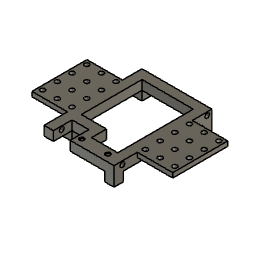
Trolley Base Assembly (Autodesk Fusion 360 design; units mm, degrees)
Autodesk Fusion 360 part; units mm, degrees
sketch "Sketch1" plane through (0, 0, 0) normal (0, 0, 1) x (1, 0, 0)
  line L0 (0, 0) -> (75, 0)
  line L1 (75, 0) -> (75, 100)
  line L2 (75, 100) -> (0, 100)
  line L3 (0, 100) -> (0, 0)
  line L4 (10, 90) -> (65, 90)
  line L5 (65, 90) -> (65, 10)
  line L6 (65, 10) -> (10, 10)
  line L7 (10, 10) -> (10, 90)
  dimension "d1" = 75
  dimension "d2" = 100
  dimension "d3" = 10
  dimension "d4" = 10
  dimension "d5" = 10
  dimension "d6" = 10
  constraint horizontal L0
  constraint vertical L1
  constraint horizontal L2
  constraint vertical L3
  constraint coincident L0.start L3.end
  constraint horizontal L4
  constraint vertical L5
  constraint horizontal L6
  constraint vertical L7
  measures "d1" distance of L1 L3
  measures "d2" distance of L0 L2
  measures "d3" distance of L0 L6
  measures "d4" distance of L1 L5
  measures "d5" distance of L2 L4
  measures "d6" distance of L3 L7
extrude "Extrude1" add sketch "Sketch1" along normal blind 10 makes body 1
sketch "Sketch2" plane through (0, 0, 0) normal (0, 0, -1) x (1, 0, 0)
  line L0 (10, -10) -> (65, -10)
  line L1 (65, -10) -> (65, -90)
  line L2 (65, -90) -> (10, -90)
  line L3 (10, -90) -> (10, -10)
  line L4 (0, 0) -> (0, -100)
  line L5 (0, -100) -> (75, -100)
  line L6 (75, -100) -> (75, 0)
  line L7 (75, 0) -> (0, 0)
  line L8 (10, -10) -> (0, -10)
  line L9 (0, -10) -> (0, 0)
  line L10 (0, 0) -> (10, 0)
  line L11 (10, 0) -> (10, -10)
  line L12 (65, -10) -> (75, -10)
  line L13 (75, -10) -> (75, 0)
  line L14 (75, 0) -> (65, 0)
  line L15 (65, 0) -> (65, -10)
  line L16 (65, -90) -> (75, -90)
  line L17 (75, -90) -> (75, -100)
  line L18 (75, -100) -> (65, -100)
  line L19 (65, -100) -> (65, -90)
  line L20 (0, -90) -> (10, -90)
  line L21 (10, -90) -> (10, -100)
  line L22 (10, -100) -> (0, -100)
  line L23 (0, -100) -> (0, -90)
  constraint horizontal L8
  constraint vertical L9
  constraint horizontal L10
  constraint vertical L11
  constraint coincident L4.start L7.end
  constraint coincident L0.start L3.end
  constraint horizontal L12
  constraint vertical L13
  constraint horizontal L14
  constraint vertical L15
  constraint coincident L6.end L7.start
  constraint coincident L0.end L1.start
  constraint horizontal L16
  constraint vertical L17
  constraint horizontal L18
  constraint vertical L19
  constraint coincident L5.end L6.start
  constraint coincident L1.end L2.start
  constraint horizontal L20
  constraint vertical L21
  constraint horizontal L22
  constraint vertical L23
  constraint coincident L5 L21.end
extrude "Extrude2" add sketch "Sketch2" along normal blind 10 contours L4 L7 L8 L9 L10 L11 | L6 L7 L12 L13 L14 L15 | L4 L5 L20 L21 L22 L23 | L5 L6 L16 L17 L18 L19 bodies 1
sketch "Sketch3" plane through (75, 0, 0) normal (1, 0, 0) x (0, 1, 0)
  line L0 (10, 0) -> (90, 0)
  line L1 (90, 0) -> (90, -10)
  line L2 (90, -10) -> (100, -10)
  line L3 (100, -10) -> (100, 10)
  line L4 (100, 10) -> (0, 10)
  line L5 (0, 10) -> (0, -10)
  line L6 (0, -10) -> (10, -10)
  line L7 (10, -10) -> (10, 0)
  circle A0 centre (5, 5) radius 2.5
  circle A1 centre (95, 5) radius 2.5
  dimension "d11" = 5
  dimension "d12" = 5
  dimension "d13" = 5
  dimension "d14" = 5
  dimension "d15" = 5
  dimension "d16" = 5
  measures "d11" diameter of A1
  measures "d12" diameter of A0
  measures "d13" distance of L4 A1.centre
  measures "d14" distance of L3 A1.centre
  measures "d15" distance of L4 A0.centre
  measures "d16" distance of L5 A0.centre
extrude "Extrude3" cut sketch "Sketch3" against normal blind 80 contours A0 | A1 bodies 1
sketch "Sketch4" plane through (0, 0, 0) normal (0, 0, -1) x (1, 0, 0)
  line L0 (10, 0) -> (10, -10)
  line L1 (10, -10) -> (65, -10)
  line L2 (65, -10) -> (65, 0)
  line L3 (65, 0) -> (10, 0)
  circle A0 centre (33, -5) radius 2.5
  circle A1 centre (61, -5) radius 2.5
  line L4 (10, -10) -> (10, -90)
  line L5 (65, -90) -> (65, -10)
  line L6 (10, -50) -> (65, -50)
  circle A2 centre (61, -95) radius 2.5
  circle A3 centre (33, -95) radius 2.5
  dimension "d19" = 5
  dimension "d20" = 23
  dimension "d21" = 5
  dimension "d22" = 4
  dimension "d23" = 5
  dimension "d24" = 5
  constraint midpoint L4 L6.start
  constraint midpoint L5 L6.end
  constraint symmetric A0 L6 A3
  constraint symmetric A1 L6 A2
  measures "d19" diameter of A0
  measures "d20" distance of L0 A0.centre
  measures "d21" diameter of A1
  measures "d22" distance of L2 A1.centre
  measures "d23" distance of L1 A1.centre
  measures "d24" diameter of A0
extrude "Extrude4" cut sketch "Sketch4" against normal blind 12 contours A0 | A1 bodies 1
extrude "Extrude5" cut sketch "Sketch4" against normal blind 12 contours A2 | A3 bodies 1
sketch "Sketch6" plane through (0, 0, 10) normal (0, 0, 1) x (-1, 0, 0)
  circle A0 centre (-33, -95) radius 2.5
  circle A1 centre (-61, -95) radius 2.5
  circle A2 centre (-33, -5) radius 2.5
  circle A3 centre (-61, -5) radius 2.5
  line L0 (-65, -10) -> (-10, -10)
  line L1 (-10, -10) -> (-10, -90)
  line L2 (-10, -90) -> (-65, -90)
  line L3 (-65, -90) -> (-65, -10)
  line L4 (0, -100) -> (0, 0)
  line L5 (0, 0) -> (-75, 0)
  line L6 (-75, 0) -> (-75, -100)
  line L7 (-75, -100) -> (0, -100)
  line L8 (-75, -80) -> (-105, -80)
  line L9 (-105, -80) -> (-105, -20)
  line L10 (-105, -20) -> (-75, -20)
  line L11 (-75, -20) -> (-75, -80)
  line L12 (-37.5, -10) -> (-37.5, -90)
  line L13 (30, -20) -> (0, -20)
  line L14 (0, -80) -> (30, -80)
  line L15 (0, -20) -> (0, -80)
  line L16 (30, -80) -> (30, -20)
  dimension "d32" = 30
  dimension "d33" = 20
  dimension "d34" = 20
  constraint horizontal L8
  constraint vertical L9
  constraint horizontal L10
  constraint vertical L11
  constraint coincident L6 L8.start
  constraint midpoint L0 L12.start
  constraint midpoint L2 L12.end
  constraint symmetric L8.start L12 L14.start
  constraint symmetric L8.end L12 L14.end
  constraint symmetric L9.end L12 L13.start
  constraint symmetric L10.end L12 L13.end
  measures "d32" distance of L9 L11
  measures "d33" distance of L5 L10
  measures "d34" distance of L7 L8
extrude "Extrude6" add sketch "Sketch6" against normal blind 5 contours L4 L13 L14 L15 L16 | L6 L8 L9 L10 L11 bodies 1
sketch "Sketch7" plane through (0, 0, 10) normal (0, 0, 1) x (-1, 0, 0)
  circle A0 centre (-33, -95) radius 2.5
  circle A1 centre (-61, -95) radius 2.5
  circle A2 centre (-33, -5) radius 2.5
  circle A3 centre (-61, -5) radius 2.5
  line L0 (-65, -10) -> (-10, -10)
  line L1 (-10, -10) -> (-10, -90)
  line L2 (-10, -90) -> (-65, -90)
  line L3 (-65, -90) -> (-65, -10)
  line L4 (0, -100) -> (0, -80)
  line L5 (0, -80) -> (30, -80)
  line L6 (30, -80) -> (30, -20)
  line L7 (30, -20) -> (0, -20)
  line L8 (0, -20) -> (0, 0)
  line L9 (0, 0) -> (-75, 0)
  line L10 (-75, 0) -> (-75, -20)
  line L11 (-75, -20) -> (-105, -20)
  line L12 (-105, -20) -> (-105, -80)
  line L13 (-105, -80) -> (-75, -80)
  line L14 (-75, -80) -> (-75, -100)
  line L15 (-75, -100) -> (0, -100)
  line L16 (0, -20) -> (-28, -20)
  line L17 (-28, -20) -> (-28, 0)
  line L18 (-28, 0) -> (0, 0)
  line L19 (0, 0) -> (0, -20)
  dimension "d37" = 28
  constraint horizontal L16
  constraint vertical L17
  constraint horizontal L18
  constraint vertical L19
  constraint coincident L9 L17.end
  constraint coincident L7.end L8.start
  measures "d37" distance of L17 L19
extrude "Extrude7" cut sketch "Sketch7" against normal blind 20 contours L0 L1 L8 L9 L16 L17 L18 L19 | L0 L1 L16 L17 bodies 1
sketch "Sketch8" plane through (0, 0, 10) normal (0, 0, 1) x (-1, 0, 0)
  line L0 (30, -20) -> (-10, -20)
  line L1 (-10, -20) -> (-10, -90)
  line L2 (-10, -90) -> (-65, -90)
  line L3 (-65, -90) -> (-65, -10)
  line L4 (-65, -10) -> (-28, -10)
  line L5 (-28, -10) -> (-28, 0)
  line L6 (-28, 0) -> (-75, 0)
  line L7 (-75, 0) -> (-75, -20)
  line L8 (-75, -20) -> (-105, -20)
  line L9 (-105, -20) -> (-105, -80)
  line L10 (-105, -80) -> (-75, -80)
  line L11 (-75, -80) -> (-75, -100)
  line L12 (-75, -100) -> (0, -100)
  line L13 (0, -100) -> (0, -80)
  line L14 (0, -80) -> (30, -80)
  line L15 (30, -80) -> (30, -20)
  circle A0 centre (-33, -95) radius 2.5
  circle A1 centre (-61, -95) radius 2.5
  circle A2 centre (-33, -5) radius 2.5
  circle A3 centre (-61, -5) radius 2.5
  line L16 (-10, -20) -> (-28, -20)
  line L17 (-36.8946, -30) -> (-10, -30)
  line L18 (-10, -30) -> (-10, -20)
  line L19 (-28, -10) -> (-36.8946, -10)
  line L20 (-36.8946, -10) -> (-36.8946, -20)
  line L21 (-28, -20) -> (-28, -10)
  line L22 (-36.8946, -20) -> (-36.8946, -30)
  dimension "d40" = 10
  constraint horizontal L16
  constraint horizontal L17
  constraint vertical L18
  constraint coincident L0.end L1.start
  constraint horizontal L19
  constraint vertical L20
  constraint vertical L21
  constraint coincident L4.end L5.start
  constraint perpendicular L17 L22
  measures "d40" distance of L16 L17
extrude "Extrude8" add sketch "Sketch8" against normal blind 10 contours L1 L4 L16 L17 L18 L19 L20 L21 L22 bodies 1
sketch "Sketch9" plane through (0, 0, 0) normal (0, 0, -1) x (1, 0, 0)
  circle A0 centre (61, -5) radius 2.5
  circle A1 centre (33, -5) radius 2.5
  line L0 (28, -20) -> (0, -20)
  line L1 (0, -20) -> (0, -90)
  line L2 (0, -90) -> (10, -90)
  line L3 (10, -90) -> (10, -30)
  line L4 (10, -30) -> (36.8946, -30)
  line L5 (36.8946, -30) -> (36.8946, -10)
  line L6 (36.8946, -10) -> (65, -10)
  line L7 (65, -10) -> (65, 0)
  line L8 (65, 0) -> (28, 0)
  line L9 (28, 0) -> (28, -20)
  line L10 (0, -20) -> (10, -20)
  line L11 (10, -20) -> (10, -30)
  line L12 (10, -30) -> (0, -30)
  line L13 (0, -30) -> (0, -20)
  constraint horizontal L10
  constraint vertical L11
  constraint horizontal L12
  constraint vertical L13
  constraint coincident L3.end L4.start
  constraint coincident L0.end L1.start
extrude "Extrude9" add sketch "Sketch9" along normal blind 10 contours L0 L1 L10 L11 L12 L13 bodies 1
sketch "Sketch10" plane through (0, 0, 10) normal (0, 0, 1) x (-1, 0, 0)
  line L0 (-10, -30) -> (-10, -90)
  line L1 (-10, -90) -> (-65, -90)
  line L2 (-65, -90) -> (-65, -10)
  line L3 (-65, -10) -> (-36.8946, -10)
  line L4 (-36.8946, -10) -> (-36.8946, -30)
  line L5 (-36.8946, -30) -> (-10, -30)
  line L6 (30, -20) -> (-28, -20)
  line L7 (-28, -20) -> (-28, 0)
  line L8 (-28, 0) -> (-75, 0)
  line L9 (-75, 0) -> (-75, -20)
  line L10 (-75, -20) -> (-105, -20)
  line L11 (-105, -20) -> (-105, -80)
  line L12 (-105, -80) -> (-75, -80)
  line L13 (-75, -80) -> (-75, -100)
  line L14 (-75, -100) -> (0, -100)
  line L15 (0, -100) -> (0, -80)
  line L16 (0, -80) -> (30, -80)
  line L17 (30, -80) -> (30, -20)
  circle A0 centre (-33, -95) radius 2.5
  circle A1 centre (-61, -95) radius 2.5
  circle A2 centre (-33, -5) radius 2.5
  circle A3 centre (-61, -5) radius 2.5
  line L18 (-30, -100) -> (-37.5, -100)
  line L19 (-37.5, -100) -> (-37.5, -90)
  line L20 (-37.5, -90) -> (-30, -90)
  line L21 (-30, -90) -> (-30, -100)
  constraint horizontal L18
  constraint vertical L19
  constraint horizontal L20
  constraint vertical L21
  constraint midpoint L1 L19.end
  constraint coincident L14 L18.start
extrude "Extrude10" add sketch "Sketch10" against normal blind 10 contours L1 L14 L18 L19 L20 L21 | A0 bodies 1
sketch "Sketch11" plane through (0, 0, 10) normal (0, 0, 1) x (-1, 0, 0)
  line L0 (-75, -100) -> (0, -100)
  line L1 (0, -100) -> (0, -80)
  line L2 (0, -80) -> (30, -80)
  line L3 (30, -80) -> (30, -20)
  line L4 (30, -20) -> (-28, -20)
  line L5 (-28, -20) -> (-28, 0)
  line L6 (-28, 0) -> (-75, 0)
  line L7 (-75, 0) -> (-75, -20)
  line L8 (-75, -20) -> (-105, -20)
  line L9 (-105, -20) -> (-105, -80)
  line L10 (-105, -80) -> (-75, -80)
  line L11 (-75, -80) -> (-75, -100)
  line L12 (-10, -90) -> (-65, -90)
  line L13 (-65, -90) -> (-65, -10)
  line L14 (-65, -10) -> (-36.8946, -10)
  line L15 (-36.8946, -10) -> (-36.8946, -30)
  line L16 (-36.8946, -30) -> (-10, -30)
  line L17 (-10, -30) -> (-10, -90)
  circle A0 centre (-61, -95) radius 2.5
  circle A1 centre (-33, -5) radius 2.5
  circle A2 centre (-61, -5) radius 2.5
  circle A3 centre (-45.25, -95) radius 2.5
  line L18 (-37.375, -90) -> (-37.375, -100)
  circle A4 centre (-29.5, -95) radius 2.5
  circle A5 centre (-13.75, -95) radius 2.5
  line L19 (-10, -87.125) -> (-65, -87.125)
  circle A6 centre (-13.75, -79.25) radius 2.5
  circle A7 centre (-29.5, -79.25) radius 2.5
  circle A8 centre (-45.25, -79.25) radius 2.5
  circle A9 centre (-61, -79.25) radius 2.5
  line L20 (-10, -71.375) -> (-65, -71.375)
  circle A10 centre (-13.75, -63.5) radius 2.5
  circle A11 centre (-13.75, -47.75) radius 2.5
  circle A12 centre (-29.5, -63.5) radius 2.5
  circle A13 centre (-29.5, -47.75) radius 2.5
  circle A14 centre (-45.25, -63.5) radius 2.5
  circle A15 centre (-61, -63.5) radius 2.5
  circle A16 centre (-61, -47.75) radius 2.5
  circle A17 centre (-45.25, -47.75) radius 2.5
  line L21 (-149.6879, -20) -> (-149.6879, -100)
  line L22 (-10, -39.875) -> (-65, -39.875)
  circle A18 centre (-13.75, -32) radius 2.5
  circle A19 centre (-29.5, -32) radius 2.5
  circle A20 centre (-45.25, -32) radius 2.5
  circle A21 centre (-61, -32) radius 2.5
  circle A22 centre (-13.75, -16.25) radius 2.5
  circle A23 centre (-285.6257, -32) radius 2.5
  circle A24 centre (-285.6257, -47.75) radius 2.5
  circle A25 centre (-269.8757, -47.75) radius 2.5
  circle A26 centre (-269.8757, -32) radius 2.5
  circle A27 centre (-269.8757, -63.5) radius 2.5
  circle A28 centre (-285.6257, -63.5) radius 2.5
  circle A29 centre (-254.1257, -32) radius 2.5
  circle A30 centre (-254.1257, -47.75) radius 2.5
  circle A31 centre (-254.1257, -63.5) radius 2.5
  line L23 (-75, 0) -> (-65, 0)
  line L24 (-65, -100) -> (-75, -100)
  line L25 (-75, -10) -> (-65, -10)
  line L26 (-68.875, -100) -> (-68.875, -10)
  circle A32 centre (-76.75, -47.75) radius 2.5
  circle A33 centre (-76.75, -32) radius 2.5
  circle A34 centre (-92.5, -32) radius 2.5
  circle A35 centre (-92.5, -63.5) radius 2.5
  circle A36 centre (-92.5, -47.75) radius 2.5
  circle A37 centre (-76.75, -63.5) radius 2.5
  circle A38 centre (-108.25, -32) radius 2.5
  circle A39 centre (-108.25, -47.75) radius 2.5
  circle A40 centre (-108.25, -63.5) radius 2.5
  circle A41 centre (-108.25, -79.25) radius 2.5
  circle A42 centre (-92.5, -79.25) radius 2.5
  circle A43 centre (-76.75, -79.25) radius 2.5
  circle A44 centre (-285.6257, -79.25) radius 2.5
  circle A45 centre (-269.8757, -79.25) radius 2.5
  circle A46 centre (-254.1257, -79.25) radius 2.5
  line L27 (-5.875, -20) -> (-5.875, -95)
  circle A47 centre (2, -79.25) radius 2.5
  circle A48 centre (17.75, -79.25) radius 2.5
  circle A49 centre (17.75, -63.5) radius 2.5
  circle A50 centre (2, -63.5) radius 2.5
  circle A51 centre (17.75, -47.75) radius 2.5
  circle A52 centre (2, -47.75) radius 2.5
  circle A53 centre (2, -32) radius 2.5
  circle A54 centre (17.75, -32) radius 2.5
  circle A55 centre (33.5, -79.25) radius 2.5
  circle A56 centre (33.5, -63.5) radius 2.5
  circle A57 centre (33.5, -47.75) radius 2.5
  circle A58 centre (33.5, -32) radius 2.5
  line L28 (0, -97.5) -> (-75, -97.5)
  line L29 (-75, -100) -> (0, -100)
  circle A59 centre (-13.75, -100) radius 2.5
  circle A60 centre (-29.5, -100) radius 2.5
  circle A61 centre (-45.25, -100) radius 2.5
  circle A62 centre (-61, -100) radius 2.5
  dimension "d48" = 15.75
  dimension "d49" = 5
  dimension "d50" = 7.875
  dimension "d51" = 7.875
  dimension "d52" = 7.875
  dimension "d53" = 7.875
  dimension "d55" = 7.875
  dimension "d75" = 7.875
  dimension "d86" = 2.5
  constraint coincident L12 L18.start
  constraint coincident L0 L18.end
  constraint perpendicular L0 L18
  constraint symmetric A0 L18 A5
  constraint symmetric A3 L18 A4
  constraint coincident L17 L19.start
  constraint coincident L13 L19.end
  constraint perpendicular L13 L19
  constraint symmetric A0 L19 A9
  constraint symmetric A3 L19 A8
  constraint symmetric A4 L19 A7
  constraint symmetric A5 L19 A6
  constraint coincident L17 L20.start
  constraint coincident L13 L20.end
  constraint perpendicular L13 L20
  constraint symmetric A0 L20 A16
  constraint symmetric A3 L20 A17
  constraint symmetric A4 L20 A13
  constraint symmetric A5 L20 A11
  constraint symmetric A6 L20 A10
  constraint symmetric A7 L20 A12
  constraint symmetric A8 L20 A14
  constraint symmetric A9 L20 A15
  constraint coincident L4 L21.start
  constraint perpendicular L4 L21
  constraint coincident L17 L22.start
  constraint coincident L13 L22.end
  constraint perpendicular L13 L22
  constraint symmetric A10 L22 A22
  constraint symmetric A11 L22 A18
  constraint symmetric A13 L22 A19
  constraint symmetric A16 L22 A21
  constraint symmetric A17 L22 A20
  constraint symmetric A10 L21 A28
  constraint symmetric A11 L21 A24
  constraint symmetric A12 L21 A27
  constraint symmetric A13 L21 A25
  constraint symmetric A14 L21 A31
  constraint symmetric A17 L21 A30
  constraint symmetric L21 A18 A23
  constraint symmetric L21 A19 A26
  constraint symmetric L21 A20 A29
  constraint coincident L24 L26.start
  constraint coincident L25 L26.end
  constraint perpendicular L14 L26
  constraint symmetric A7 L26 A41
  constraint symmetric A8 L26 A42
  constraint symmetric A9 L26 A43
  constraint symmetric A12 L26 A40
  constraint symmetric A13 L26 A39
  constraint symmetric A14 L26 A35
  constraint symmetric A15 L26 A37
  constraint symmetric A16 L26 A32
  constraint symmetric A17 L26 A36
  constraint symmetric A19 L26 A38
  constraint symmetric A20 L26 A34
  constraint symmetric A21 L26 A33
  constraint symmetric A6 L21 A44
  constraint symmetric A7 L21 A45
  constraint symmetric A8 L21 A46
  constraint coincident L4 L27.start
  constraint perpendicular L4 L27
  constraint symmetric A6 L27 A47
  constraint symmetric A7 L27 A48
  constraint symmetric A8 L27 A55
  constraint symmetric A10 L27 A50
  constraint symmetric A11 L27 A52
  constraint symmetric A12 L27 A49
  constraint symmetric A13 L27 A51
  constraint symmetric A14 L27 A56
  constraint symmetric A17 L27 A57
  constraint symmetric A18 L27 A53
  constraint symmetric A19 L27 A54
  constraint symmetric A20 L27 A58
  constraint coincident L1 L28.start
  constraint coincident L11 L28.end
  constraint perpendicular L11 L28
  constraint symmetric A0 L28 A62
  constraint symmetric A3 L28 A61
  constraint symmetric A4 L28 A60
  constraint symmetric A5 L28 A59
  measures "d48" distance of A0.centre A3.centre
  measures "d49" diameter of A3
  measures "d50" distance of A3.centre L18
  measures "d51" distance of A4.centre L19
  measures "d52" distance of A7.centre L20
  measures "d53" distance of A13.centre L22
  measures "d55" distance of A16.centre L26
  measures "d75" distance of A6.centre L27
  measures "d86" distance of L28 L29
sketch "Sketch12" plane through (0, 0, 10) normal (0, 0, 1) x (-1, 0, 0)
  line L0 (-105, -20) -> (-113, -20)
  line L1 (-113, -20) -> (-113, -84)
  line L2 (-113, -84) -> (-105, -84)
  line L3 (-105, -84) -> (-105, -20)
  line L4 (-105, -80) -> (-75, -80)
  line L5 (-105, -84) -> (-75, -84)
  line L6 (-75, -84) -> (-75, -80)
  line L7 (-75, -80) -> (-105, -80)
  line L8 (-105, -80) -> (-105, -84)
  line L9 (-113, -20) -> (-75, -20)
  line L10 (-75, -20) -> (-75, -25)
  line L11 (-75, -25) -> (-113, -25)
  line L12 (-113, -25) -> (-113, -20)
  line L13 (-75, -80) -> (-75, -20)
  line L14 (30, -20) -> (38, -20)
  line L15 (38, -20) -> (38, -84)
  line L16 (38, -84) -> (30, -84)
  line L17 (30, -84) -> (30, -20)
  line L18 (0, -80) -> (30, -80)
  line L19 (30, -84) -> (0, -84)
  line L20 (0, -84) -> (0, -80)
  line L21 (0, -80) -> (30, -80)
  line L22 (30, -80) -> (30, -84)
  line L23 (38, -20) -> (0, -20)
  line L24 (0, -20) -> (0, -25)
  line L25 (0, -25) -> (38, -25)
  line L26 (38, -25) -> (38, -20)
  line L27 (0, -20) -> (0, -30)
  point P0 (-105, -20)
  point P1 (30, -20)
  dimension "d56" = 8
  dimension "d57" = 4
  dimension "d58" = 8
  dimension "d59" = 4
  dimension "d60" = 5
  constraint horizontal L0
  constraint vertical L1
  constraint horizontal L2
  constraint vertical L3
  constraint coincident P0 L0.start
  constraint horizontal L5
  constraint vertical L6
  constraint horizontal L7
  constraint vertical L8
  constraint coincident L4.end L6.end
  constraint horizontal L9
  constraint vertical L10
  constraint horizontal L11
  constraint vertical L12
  constraint coincident L10.end L13
  constraint horizontal L14
  constraint vertical L15
  constraint horizontal L16
  constraint vertical L17
  constraint coincident P1 L14.start
  constraint horizontal L19
  constraint vertical L20
  constraint horizontal L21
  constraint vertical L22
  constraint coincident L18.start L20.end
  constraint horizontal L23
  constraint vertical L24
  constraint horizontal L25
  constraint vertical L26
  constraint midpoint L24.end L27
  measures "d56" distance of L1 L3
  measures "d57" distance of L2 L4
  measures "d58" distance of L15 L17
  measures "d59" distance of L16 L18
  measures "d60" distance of L23 L25
extrude "Extrude11" add sketch "Sketch12" against normal blind 5 contours L1 L2 L3 L8 L11 | L3 L4 L5 L6 L7 L8 bodies 1
extrude "Extrude12" cut sketch "Sketch12" against normal blind 5 contours L0 L1 L3 L9 L11 L12 | L3 L9 L10 L11 L13 bodies 1
extrude "Extrude13" add sketch "Sketch12" against normal blind 5 contours L15 L16 L17 L22 L25 | L17 L18 L19 L20 L21 L22 bodies 1
extrude "Extrude14" cut sketch "Sketch12" against normal blind 5 contours L14 L15 L17 L23 L25 L26 | L17 L23 L24 L25 L27 bodies 1
extrude "Extrude15" cut sketch "Sketch11" against normal blind 10 contours A3 | A4 | A5 bodies 1
extrude "Extrude16" cut sketch "Sketch11" against normal blind 10 contours L10 L11 A43 | L10 L11 A43 | A32 | A33 | A37 bodies 1
extrude "Extrude17" cut sketch "Sketch11" against normal blind 5 contours L10 A42 | L10 A42 | A34 | A35 | A36 | A38 | A39 | A40 | A41 bodies 1
extrude "Extrude18" cut sketch "Sketch11" against normal blind 10 contours L1 L2 A47 | L1 L2 A47 | L2 A48 | L2 A48 | A49 | A50 | A51 | A52 | A53 | A54 | A55 | A56 | A57 | A58 bodies 1
sketch "Sketch13" plane through (75, 0, 0) normal (1, 0, 0) x (0, 1, 0)
  circle A0 centre (95, 5) radius 2.5
  line L0 (81.0354, 5) -> (81.0354, 0)
  line L1 (81.0354, 0) -> (90, 0)
  line L2 (90, 0) -> (90, -10)
  line L3 (90, -10) -> (100, -10)
  line L4 (100, -10) -> (100, 10)
  line L5 (100, 10) -> (84, 10)
  line L6 (84, 10) -> (84, 5)
  line L7 (84, 5) -> (81.0354, 5)
  circle A1 centre (95, 5) radius 2.5
  constraint concentric A0 A1
extrude "Extrude19" cut 1 faces at (37.5, 95.4167, 5.8298) along direction (1, 0, 0) blind -500 and the other way blind -500 on bodies 1 bodies 1
sketch "Sketch14" plane through (0, 20, 0) normal (0, -1, 0) x (1, 0, 0)
  line L0 (0, 10) -> (0, -10)
  line L1 (0, -10) -> (10, -10)
  line L2 (10, -10) -> (10, 0)
  line L3 (10, 0) -> (28, 0)
  line L4 (28, 0) -> (28, 10)
  line L5 (28, 10) -> (0, 10)
  line L6 (10, 0) -> (0, 0)
  line L7 (0, 0) -> (0, 10)
  line L8 (0, 10) -> (10, 10)
  line L9 (10, 10) -> (10, 0)
  constraint horizontal L6
  constraint vertical L7
  constraint horizontal L8
  constraint vertical L9
  constraint coincident L0.start L5.end
  constraint coincident L2.end L3.start
extrude "Extrude20" add sketch "Sketch14" along normal blind 20 contours L0 L5 L6 L7 L8 L9 bodies 1
sketch "Sketch15" plane through (28, 0, 0) normal (-1, 0, 0) x (0, -1, 0)
  line L0 (-20, 0) -> (0, 0)
  line L1 (0, 0) -> (0, 10)
  line L2 (0, 10) -> (-20, 10)
  line L3 (-20, 10) -> (-20, 0)
  circle A0 centre (-5, 5) radius 2.5
sketch "Sketch16" plane through (75, 0, 0) normal (1, 0, 0) x (0, 1, 0)
  line L0 (30.2146, 0) -> (30.2146, 5)
  line L1 (30.2146, 5) -> (25, 5)
  line L2 (25, 5) -> (25, 10)
  line L3 (25, 10) -> (0, 10)
  line L4 (0, 10) -> (0, -10)
  line L5 (0, -10) -> (10, -10)
  line L6 (10, -10) -> (10, 0)
  line L7 (10, 0) -> (30.2146, 0)
  circle A0 centre (5, 5) radius 2.5
  circle A1 centre (5, 5) radius 2.5
  constraint concentric A0 A1
extrude "Extrude21" cut sketch "Sketch16" against normal blind 500 contours A0 A1 bodies 1
sketch "Sketch17" plane through (0, 0, 0) normal (-1, 0, 0) x (0, -1, 0)
  circle A0 centre (-95, 5) radius 2.5
  line L0 (-80.75, 0) -> (-80.75, 5)
  line L1 (-80.75, 5) -> (-84, 5)
  line L2 (-84, 5) -> (-84, 10)
  line L3 (-84, 10) -> (-100, 10)
  line L4 (-100, 10) -> (-100, -10)
  line L5 (-100, -10) -> (-90, -10)
  line L6 (-90, -10) -> (-90, 0)
  line L7 (-90, 0) -> (-80.75, 0)
sketch "Sketch18" plane through (75, 0, 0) normal (1, 0, 0) x (0, 1, 0)
  circle A0 centre (95, 5) radius 2.5
  line L0 (81.0354, 5) -> (81.0354, 0)
  line L1 (81.0354, 0) -> (90, 0)
  line L2 (90, 0) -> (90, -10)
  line L3 (90, -10) -> (100, -10)
  line L4 (100, -10) -> (100, 10)
  line L5 (100, 10) -> (84, 10)
  line L6 (84, 10) -> (84, 5)
  line L7 (84, 5) -> (81.0354, 5)
  line L8 (90, 0) -> (100, 0)
  line L9 (97.5, 0) -> (97.5, 10)
  line L10 (100, -10) -> (100, 10)
  circle A1 centre (100, 5) radius 2.5
  line L11 (90, 0) -> (100, 0)
  line L12 (100, 0) -> (100, 10)
  line L13 (100, 10) -> (90, 10)
  line L14 (90, 10) -> (90, 0)
  line L15 (90, 0) -> (100, 0)
  line L16 (100, 0) -> (100, -10)
  line L17 (100, -10) -> (90, -10)
  line L18 (90, -10) -> (90, 0)
  line L19 (100, 10) -> (100, 0)
  line L20 (100, -10) -> (100, 0)
  line L21 (90, 10) -> (100, 10)
  line L22 (100, 10) -> (100, 0)
  line L23 (100, 0) -> (90, 0)
  line L24 (90, 0) -> (90, 10)
  line L25 (100, 10) -> (105, 10)
  line L26 (105, 10) -> (105, 0)
  line L27 (105, 0) -> (100, 0)
  line L28 (100, 0) -> (100, 10)
  line L29 (100, 0) -> (105, 0)
  line L30 (105, 0) -> (105, -10)
  line L31 (105, -10) -> (100, -10)
  line L32 (100, -10) -> (100, 0)
  line L33 (90, 0) -> (95, 0)
  line L34 (95, 0) -> (95, -10)
  line L35 (95, -10) -> (90, -10)
  line L36 (90, -10) -> (90, 0)
  dimension "d87" = 2.5
  constraint coincident L8 L9.start
  constraint coincident L5 L9.end
  constraint symmetric A0 L9 A1
  constraint horizontal L11
  constraint vertical L12
  constraint horizontal L13
  constraint vertical L14
  constraint coincident L4.end L5.start
  constraint coincident L1.end L2.start
  constraint horizontal L15
  constraint vertical L16
  constraint horizontal L17
  constraint vertical L18
  constraint coincident L3.end L4.start
  constraint vertical L19
  constraint vertical L20
  constraint horizontal L21
  constraint vertical L22
  constraint horizontal L23
  constraint vertical L24
  constraint horizontal L25
  constraint vertical L26
  constraint horizontal L27
  constraint vertical L28
  constraint horizontal L29
  constraint vertical L30
  constraint horizontal L31
  constraint vertical L32
  constraint horizontal L33
  constraint vertical L34
  constraint horizontal L35
  constraint vertical L36
  constraint midpoint L3 L34.end
  measures "d87" distance of L9 L10
extrude "Extrude22" add sketch "Sketch18" against normal blind 75 contours L4 L10 A1 L12 L19 L22 L28 | L4 L10 A1 L12 L19 L22 L25 L26 L27 L28 L29 picked at (100.8333, 5) bodies 1
extrude "Extrude23" add sketch "Sketch18" against normal blind 75 contours L4 L10 L16 L20 L27 L29 L30 L31 L32 bodies 1
extrude "Extrude24" cut sketch "Sketch18" against normal blind 75 contours L2 L3 L8 L11 L15 L17 L18 L23 L33 L34 L35 L36 bodies 1
sketch "Sketch19" plane through (0, 105, 0) normal (0, 1, 0) x (-1, 0, 0)
  line L0 (-75, 10) -> (-75, -10)
  line L1 (-75, -10) -> (0, -10)
  line L2 (0, -10) -> (0, 10)
  line L3 (0, 10) -> (-75, 10)
  line L4 (-65, -10) -> (-10, -10)
  line L5 (-10, -10) -> (-10, 0)
  line L6 (-10, 0) -> (-65, 0)
  line L7 (-65, 0) -> (-65, -10)
  point P0 (-65, -10)
  point P1 (-10, 0)
  constraint horizontal L4
  constraint vertical L5
  constraint horizontal L6
  constraint vertical L7
  constraint coincident P1 L5.end
  constraint coincident P0 L4.start
extrude "Extrude25" cut sketch "Sketch19" against normal blind 10 contours L1 L4 L5 L6 L7 bodies 1
extrude "Extrude26" cut sketch "Sketch18" against normal blind 75 contours L4 L10 A1 L12 L19 L22 L28 | L4 L10 A1 L12 L19 L22 L28 bodies 1
extrude "Extrude27" add sketch "Sketch18" against normal blind 75 separate body contours A0 makes body 2
extrude "Extrude28" cut sketch "Sketch11" against normal blind 10 contours A0 | A3 | A4 | A5 bodies 2
sketch "Sketch20" plane through (75, 0, 0) normal (1, 0, 0) x (0, 1, 0)
  circle A0 centre (95, 5) radius 2.5
  circle A1 centre (95, 5) radius 2.5
  constraint concentric A0 A1
extrude "Extrude29" add sketch "Sketch20" against normal blind 75 bodies 2 1
sketch "Sketch21" plane through (0, 0, 0) normal (0, 1, 0) x (1, 0, 0)
sketch "Sketch22" plane through (0, 0, 10) normal (0, 0, 1) x (-1, 0, 0)
  circle A0 centre (17.75, -63.5) radius 2.5
  circle A1 centre (17.75, -47.75) radius 2.5
  circle A2 centre (33.5, -63.5) radius 2.5
  circle A3 centre (33.5, -47.75) radius 2.5
  circle A4 centre (2, -32) radius 2.5
  circle A5 centre (17.75, -79.25) radius 2.5
  circle A6 centre (2, -63.5) radius 2.5
  circle A7 centre (17.75, -32) radius 2.5
  circle A8 centre (33.5, -79.25) radius 2.5
  circle A9 centre (33.5, -32) radius 2.5
  circle A10 centre (2, -47.75) radius 2.5
  circle A11 centre (2, -79.25) radius 2.5
  circle A12 centre (-108.25, -32) radius 2.5
  circle A13 centre (-92.5, -32) radius 2.5
  circle A14 centre (-92.5, -63.5) radius 2.5
  circle A15 centre (-108.25, -79.25) radius 2.5
  circle A16 centre (-108.25, -47.75) radius 2.5
  circle A17 centre (-92.5, -47.75) radius 2.5
  circle A18 centre (-92.5, -79.25) radius 2.5
  circle A19 centre (-108.25, -63.5) radius 2.5
  circle A20 centre (-76.75, -47.75) radius 2.5
  circle A21 centre (-76.75, -63.5) radius 2.5
  circle A22 centre (-76.75, -32) radius 2.5
  circle A23 centre (-76.75, -79.25) radius 2.5
  circle A24 centre (-45.25, -95) radius 2.5
  circle A25 centre (-29.5, -95) radius 2.5
  circle A26 centre (-13.75, -95) radius 2.5
  line L0 (38, -25) -> (0, -25)
  line L1 (0, -25) -> (0, 0)
  line L2 (0, 0) -> (-10, 0)
  line L3 (-10, 0) -> (-10, -20)
  line L4 (-10, -20) -> (-28, -20)
  line L5 (-28, -20) -> (-28, 0)
  line L6 (-28, 0) -> (-75, 0)
  line L7 (-75, 0) -> (-75, -25)
  line L8 (-75, -25) -> (-113, -25)
  line L9 (-113, -25) -> (-113, -84)
  line L10 (-113, -84) -> (-75, -84)
  line L11 (-75, -84) -> (-75, -105)
  line L12 (-75, -105) -> (0, -105)
  line L13 (0, -105) -> (0, -84)
  line L14 (0, -84) -> (38, -84)
  line L15 (38, -84) -> (38, -25)
  line L16 (-10, -90) -> (-65, -90)
  line L17 (-65, -90) -> (-65, -10)
  line L18 (-65, -10) -> (-36.8946, -10)
  line L19 (-36.8946, -10) -> (-36.8946, -30)
  line L20 (-36.8946, -30) -> (-10, -30)
  line L21 (-10, -30) -> (-10, -90)
  circle A27 centre (-61, -95) radius 2.5
  circle A28 centre (-33, -5) radius 2.5
  circle A29 centre (-61, -5) radius 2.5
  line L22 (-28, -6.25) -> (-75, -6.25)
  circle A30 centre (-33, -7.5) radius 2.5
  circle A31 centre (-61, -7.5) radius 2.5
  dimension "d104" = 1.25
  constraint coincident L5 L22.start
  constraint coincident L7 L22.end
  constraint perpendicular L7 L22
  constraint symmetric A28 L22 A30
  constraint symmetric A29 L22 A31
  measures "d104" distance of A28.centre L22
extrude "Extrude30" add sketch "Sketch22" against normal blind 10 contours A28 A30 | A28 L22 | L22 A30 picked at (-33.2804, -4.1907) bodies 2
extrude "Extrude31" add sketch "Sketch22" against normal blind 10 contours A29 A31 | A29 L22 | L22 A31 picked at (-61.2804, -4.1907) bodies 2
sketch "Sketch23" plane through (0, 0, 0) normal (-1, 0, 0) x (0, -1, 0)
  circle A0 centre (-5, 5) radius 2.5
  line L0 (-30.5, 5) -> (-30.5, 0)
  line L1 (-30.5, 0) -> (-30, 0)
  line L2 (-30, 0) -> (-30, -10)
  line L3 (-30, -10) -> (-20, -10)
  line L4 (-20, -10) -> (-20, 0)
  line L5 (-20, 0) -> (0, 0)
  line L6 (0, 0) -> (0, 10)
  line L7 (0, 10) -> (-25, 10)
  line L8 (-25, 10) -> (-25, 5)
  line L9 (-25, 5) -> (-30.5, 5)
  line L10 (-7, 0) -> (-7, 10)
  circle A1 centre (-9, 5) radius 2.5
  line L11 (0, 5.75) -> (-15, 5.75)
  circle A2 centre (-9, 6.5) radius 2.5
  dimension "d109" = 2
  dimension "d110" = 0.75
  constraint coincident L5 L10.start
  constraint coincident L7 L10.end
  constraint symmetric A0 L10 A1
  constraint coincident L6 L11.start
  constraint perpendicular L6 L11
  constraint symmetric A1 L11 A2
  measures "d109" distance of A0.centre L10
  measures "d110" distance of A1.centre L11
extrude "Extrude32" add sketch "Sketch23" against normal blind 75 contours A0 A1 L11 | A0 L11 A2 | A0 L10 A2 | L10 A1 A2 | A0 A1 A2 | L10 A1 L11 | L10 L11 A2 | A0 L10 L11 A2 | A0 L10 L11 picked at (-3.8423, 4.878) picked at (-3.9943, 5.8649) picked at (-7.0525, 4.0791) picked at (-6.6736, 4.893) picked at (-6.7351, 6.4779) bodies 2
sketch "Sketch24" plane through (0, 0, 10) normal (0, 0, 1) x (-1, 0, 0)
  circle A0 centre (17.75, -63.5) radius 2.5
  circle A1 centre (17.75, -47.75) radius 2.5
  circle A2 centre (33.5, -63.5) radius 2.5
  circle A3 centre (33.5, -47.75) radius 2.5
  circle A4 centre (2, -32) radius 2.5
  circle A5 centre (17.75, -79.25) radius 2.5
  circle A6 centre (2, -63.5) radius 2.5
  circle A7 centre (17.75, -32) radius 2.5
  circle A8 centre (33.5, -79.25) radius 2.5
  circle A9 centre (33.5, -32) radius 2.5
  circle A10 centre (2, -47.75) radius 2.5
  circle A11 centre (2, -79.25) radius 2.5
  circle A12 centre (-108.25, -32) radius 2.5
  circle A13 centre (-92.5, -32) radius 2.5
  circle A14 centre (-92.5, -63.5) radius 2.5
  circle A15 centre (-108.25, -79.25) radius 2.5
  circle A16 centre (-108.25, -47.75) radius 2.5
  circle A17 centre (-92.5, -47.75) radius 2.5
  circle A18 centre (-92.5, -79.25) radius 2.5
  circle A19 centre (-108.25, -63.5) radius 2.5
  circle A20 centre (-76.75, -47.75) radius 2.5
  circle A21 centre (-76.75, -63.5) radius 2.5
  circle A22 centre (-76.75, -32) radius 2.5
  circle A23 centre (-76.75, -79.25) radius 2.5
  circle A24 centre (-45.25, -95) radius 2.5
  circle A25 centre (-29.5, -95) radius 2.5
  circle A26 centre (-13.75, -95) radius 2.5
  line L0 (38, -25) -> (0, -25)
  line L1 (0, -25) -> (0, 0)
  line L2 (0, 0) -> (-10, 0)
  line L3 (-10, 0) -> (-10, -20)
  line L4 (-10, -20) -> (-28, -20)
  line L5 (-28, -20) -> (-28, 0)
  line L6 (-28, 0) -> (-75, 0)
  line L7 (-75, 0) -> (-75, -25)
  line L8 (-75, -25) -> (-113, -25)
  line L9 (-113, -25) -> (-113, -84)
  line L10 (-113, -84) -> (-75, -84)
  line L11 (-75, -84) -> (-75, -105)
  line L12 (-75, -105) -> (0, -105)
  line L13 (0, -105) -> (0, -84)
  line L14 (0, -84) -> (38, -84)
  line L15 (38, -84) -> (38, -25)
  line L16 (-10, -90) -> (-65, -90)
  line L17 (-65, -90) -> (-65, -10)
  line L18 (-65, -10) -> (-36.8946, -10)
  line L19 (-36.8946, -10) -> (-36.8946, -30)
  line L20 (-36.8946, -30) -> (-10, -30)
  line L21 (-10, -30) -> (-10, -90)
  circle A27 centre (-61, -95) radius 2.5
  line L22 (-36.8946, -10) -> (-65, -10)
  line L23 (-65, -10) -> (-65, -14)
  line L24 (-65, -14) -> (-36.8946, -14)
  line L25 (-36.8946, -14) -> (-36.8946, -10)
  line L26 (-10, -20) -> (-28, -20)
  line L27 (-28, -20) -> (-28, 0)
  line L28 (-28, 0) -> (-10, 0)
  line L29 (-10, 0) -> (-10, -20)
  dimension "d113" = 4
  constraint horizontal L22
  constraint vertical L23
  constraint horizontal L24
  constraint vertical L25
  constraint coincident L17 L23.end
  constraint coincident L18.end L19.start
  constraint horizontal L26
  constraint vertical L27
  constraint horizontal L28
  constraint vertical L29
  constraint coincident L5.end L6.start
  constraint coincident L3.end L4.start
  measures "d113" distance of L22 L24
extrude "Extrude33" add sketch "Sketch24" against normal blind 10 contours L17 L18 L19 L22 L23 L24 L25 bodies 2
extrude "Extrude34" cut sketch "Sketch24" against normal blind 10 contours L3 L4 L5 L26 L27 L28 L29 bodies 2
extrude "Extrude35" cut sketch "Sketch23" against normal blind 75 contours A0 A1 A2 | A0 L10 A2 | L10 A1 L11 | L10 L11 A2 | A0 L11 A2 | A0 L10 L11 A2 | L10 A1 A2 | A0 A1 L11 | A0 L10 L11 picked at (-6.7351, 6.4779) picked at (-6.9475, 7.4209) picked at (-10.0057, 5.6351) picked at (-8.7661, 8.4833) picked at (-10.0066, 5.8632) bodies 2
sketch "Sketch25" plane through (75, 0, 0) normal (1, 0, 0) x (0, 1, 0)
  circle A0 centre (100, 5) radius 2.5
  line L0 (95, 0) -> (95, -10)
  line L1 (95, -10) -> (105, -10)
  line L2 (105, -10) -> (105, 10)
  line L3 (105, 10) -> (84, 10)
  line L4 (84, 10) -> (84, 5)
  line L5 (84, 5) -> (81.0354, 5)
  line L6 (81.0354, 5) -> (81.0354, 0)
  line L7 (81.0354, 0) -> (95, 0)
  line L8 (105, 5.75) -> (96, 5.75)
  circle A1 centre (100, 6.5) radius 2.5
  dimension "d120" = 0.75
  constraint coincident L2 L8.start
  constraint perpendicular L2 L8
  constraint symmetric A0 L8 A1
  measures "d120" distance of A0.centre L8
extrude "Extrude36" add sketch "Sketch25" against normal blind 75 contours A0 A1 | A0 L8 | L8 A1 picked at (99.6858, 3.0262) bodies 2
extrude "Extrude37" cut sketch "Sketch25" against normal blind 75 contours A0 L8 | L8 A1 | A0 A1 picked at (99.6858, 8.4738) bodies 2
extrude "Extrude38" cut sketch "Sketch11" against normal blind 10 contours A0 | A3 | A4 | A5 bodies 2
extrude "Extrude39" cut sketch "Sketch22" against normal blind 10 contours A28 A30 | A28 L22 | L22 A30 | A29 A31 | A29 L22 | L22 A31 picked at (-33.2804, -8.3093) picked at (-61.3698, -9.1203) bodies 2
sketch "Sketch26" plane through (0, 0, 10) normal (0, 0, 1) x (-1, 0, 0)
  circle A0 centre (-33, -7.5) radius 2.5
  circle A1 centre (-61, -7.5) radius 2.5
  circle A2 centre (17.75, -63.5) radius 2.5
  circle A3 centre (17.75, -47.75) radius 2.5
  circle A4 centre (33.5, -63.5) radius 2.5
  circle A5 centre (33.5, -47.75) radius 2.5
  circle A6 centre (2, -32) radius 2.5
  circle A7 centre (17.75, -79.25) radius 2.5
  circle A8 centre (2, -63.5) radius 2.5
  circle A9 centre (17.75, -32) radius 2.5
  circle A10 centre (33.5, -79.25) radius 2.5
  circle A11 centre (33.5, -32) radius 2.5
  circle A12 centre (2, -47.75) radius 2.5
  circle A13 centre (2, -79.25) radius 2.5
  circle A14 centre (-108.25, -32) radius 2.5
  circle A15 centre (-92.5, -32) radius 2.5
  circle A16 centre (-92.5, -63.5) radius 2.5
  circle A17 centre (-108.25, -79.25) radius 2.5
  circle A18 centre (-108.25, -47.75) radius 2.5
  circle A19 centre (-92.5, -47.75) radius 2.5
  circle A20 centre (-92.5, -79.25) radius 2.5
  circle A21 centre (-108.25, -63.5) radius 2.5
  circle A22 centre (-76.75, -47.75) radius 2.5
  circle A23 centre (-76.75, -63.5) radius 2.5
  circle A24 centre (-76.75, -32) radius 2.5
  circle A25 centre (-76.75, -79.25) radius 2.5
  circle A26 centre (-45.25, -95) radius 2.5
  circle A27 centre (-29.5, -95) radius 2.5
  circle A28 centre (-13.75, -95) radius 2.5
  line L0 (38, -25) -> (0, -25)
  line L1 (0, -25) -> (0, 0)
  line L2 (0, 0) -> (-10, 0)
  line L3 (-10, 0) -> (-10, -20)
  line L4 (-10, -20) -> (-28, -20)
  line L5 (-28, -20) -> (-28, 0)
  line L6 (-28, 0) -> (-75, 0)
  line L7 (-75, 0) -> (-75, -25)
  line L8 (-75, -25) -> (-113, -25)
  line L9 (-113, -25) -> (-113, -84)
  line L10 (-113, -84) -> (-75, -84)
  line L11 (-75, -84) -> (-75, -105)
  line L12 (-75, -105) -> (0, -105)
  line L13 (0, -105) -> (0, -84)
  line L14 (0, -84) -> (38, -84)
  line L15 (38, -84) -> (38, -25)
  line L16 (-10, -90) -> (-65, -90)
  line L17 (-65, -90) -> (-65, -14)
  line L18 (-65, -14) -> (-36.8946, -14)
  line L19 (-36.8946, -14) -> (-36.8946, -30)
  line L20 (-36.8946, -30) -> (-10, -30)
  line L21 (-10, -30) -> (-10, -90)
  circle A29 centre (-61, -95) radius 2.5
  line L22 (-10, -90) -> (-65, -90)
  line L23 (-65, -90) -> (-65, -95)
  line L24 (-65, -95) -> (-10, -95)
  line L25 (-10, -95) -> (-10, -90)
  line L26 (-65, -105) -> (-65, -95)
  dimension "d129" = 5
  constraint horizontal L22
  constraint vertical L23
  constraint horizontal L24
  constraint vertical L25
  constraint coincident L23.end L26
  constraint coincident L16.start L21.end
  measures "d129" distance of L22 L24
extrude "Extrude40" cut sketch "Sketch26" against normal blind 10 contours A26 L24 | A26 A27 A28 L16 A29 L22 L23 L24 L25 | A27 L24 | A29 L24 | A28 L24 picked at (-44.7304, -93.6253) picked at (-28.9804, -93.6253) picked at (-60.4804, -93.6253) picked at (-13.2304, -93.6253) bodies 2
sketch "Sketch27" plane through (0, 0, 10) normal (0, 0, 1) x (-1, 0, 0)
  line L0 (38, -25) -> (0, -25)
  line L1 (0, -25) -> (0, 0)
  line L2 (0, 0) -> (-10, 0)
  line L3 (-10, 0) -> (-10, -20)
  line L4 (-10, -20) -> (-28, -20)
  line L5 (-28, -20) -> (-28, 0)
  line L6 (-28, 0) -> (-75, 0)
  line L7 (-75, 0) -> (-75, -25)
  line L8 (-75, -25) -> (-113, -25)
  line L9 (-113, -25) -> (-113, -84)
  line L10 (-113, -84) -> (-75, -84)
  line L11 (-75, -84) -> (-75, -105)
  line L12 (-75, -105) -> (0, -105)
  line L13 (0, -105) -> (0, -84)
  line L14 (0, -84) -> (38, -84)
  line L15 (38, -84) -> (38, -25)
  circle A0 centre (-76.75, -79.25) radius 2.5
  circle A1 centre (-76.75, -32) radius 2.5
  circle A2 centre (-76.75, -63.5) radius 2.5
  circle A3 centre (-76.75, -47.75) radius 2.5
  circle A4 centre (-108.25, -63.5) radius 2.5
  circle A5 centre (-92.5, -79.25) radius 2.5
  circle A6 centre (-92.5, -47.75) radius 2.5
  circle A7 centre (-108.25, -47.75) radius 2.5
  circle A8 centre (-108.25, -79.25) radius 2.5
  circle A9 centre (-92.5, -63.5) radius 2.5
  circle A10 centre (-92.5, -32) radius 2.5
  circle A11 centre (-108.25, -32) radius 2.5
  circle A12 centre (2, -79.25) radius 2.5
  circle A13 centre (2, -47.75) radius 2.5
  circle A14 centre (33.5, -32) radius 2.5
  circle A15 centre (33.5, -79.25) radius 2.5
  circle A16 centre (17.75, -32) radius 2.5
  circle A17 centre (2, -63.5) radius 2.5
  circle A18 centre (17.75, -79.25) radius 2.5
  circle A19 centre (2, -32) radius 2.5
  circle A20 centre (33.5, -47.75) radius 2.5
  circle A21 centre (33.5, -63.5) radius 2.5
  circle A22 centre (17.75, -47.75) radius 2.5
  circle A23 centre (17.75, -63.5) radius 2.5
  circle A24 centre (-61, -7.5) radius 2.5
  circle A25 centre (-33, -7.5) radius 2.5
  line L16 (-16.25, -95) -> (-27, -95)
  arc A26 (-32, -95) -> (-27, -95) centre (-29.5, -95) ccw
  line L17 (-32, -95) -> (-42.75, -95)
  arc A27 (-47.75, -95) -> (-42.75, -95) centre (-45.25, -95) ccw
  line L18 (-47.75, -95) -> (-58.5, -95)
  arc A28 (-63.5, -95) -> (-58.5, -95) centre (-61, -95) ccw
  line L19 (-63.5, -95) -> (-65, -95)
  line L20 (-65, -95) -> (-65, -14)
  line L21 (-65, -14) -> (-36.8946, -14)
  line L22 (-36.8946, -14) -> (-36.8946, -30)
  line L23 (-36.8946, -30) -> (-10, -30)
  line L24 (-10, -30) -> (-10, -95)
  line L25 (-10, -95) -> (-11.25, -95)
  arc A29 (-16.25, -95) -> (-11.25, -95) centre (-13.75, -95) ccw
  line L26 (-10, -95) -> (-65, -95)
  line L27 (-65, -95) -> (-65, -97.5192)
  line L28 (-65, -97.5192) -> (-10, -97.5192)
  line L29 (-10, -97.5192) -> (-10, -95)
  line L30 (-65, -105) -> (-65, -95)
  constraint horizontal L26
  constraint vertical L27
  constraint horizontal L28
  constraint vertical L29
  constraint coincident L27.end L30
  constraint coincident L24.end L25.start
extrude "Extrude41" add sketch "Sketch27" against normal blind 10 contours A29 L26 | A26 L26 | A27 L26 | A28 L26 bodies 2
